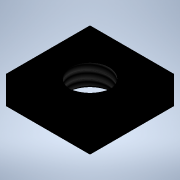
# Autodesk Inventor part: 14122
Saved by Autodesk Inventor 2021 (Build 250183000, 183)
## iProperties
Part Number: 14122
Material: Generic
Catalog Web Link: www.cadenas.de
Description: 14122-Nut
Vendor: 8020
Document SubType Name: Modeling
Designer: partserver
Manufacturer: 8020
Mass: 0.200128 g
Surface Area: 2.76017 cm^2
Volume: 0.200128 cm^3
Density: 1 g/cm^3
Appearance: PSOLRGB-0-0-0
Category: PARTsolutions
Company: 8020
PSOL_IDENT_0: {$CADENAS_DATA\23d-libs\8020\metric\fastening_options\14122.prj},149 {VTYP=3D},{NB=14122},{LINA=1412
PSOL_IDENT_1: 2},{NN=14122},{DATE=31.07.2020 09:21:26},{GEOMDATE=30.03.2012 07:06:00},{VERSION=},{LINEID=10},{WBVA
PSOL_IDENT_2: R=},{WBNUMERIC=}  {NB=14122},{LINA=14122},{KT=DUMMY},{PN=14122},{A=9.000},{B=3.000},{M=5.000}
NB: 14122
NN: 14122
NT: Nut
NBSYN: $PN.
LINA: 14122
CATALOG: 80/20
PN: 14122
A: 9
B: 3
M: 5
SUPPLIER: 8020
ARTICLENO: 14122
BOMINFO: 14122
CREATOR: CADENAS GmbH
Title: 14122
Author: Cadenas PARTsolutions
Comments: Nut
Autodesk Inventor part; units mm, degrees
sketch "Sketch_1" plane through (0, 0, 0) normal (0, 0, 1) x (1, 0, 0)
  line L0 (-4.5, 4.5) -> (-4.5, -4.5)
  line L1 (-4.5, -4.5) -> (4.5, -4.5)
  line L2 (4.5, -4.5) -> (4.5, 4.5)
  line L3 (4.5, 4.5) -> (-4.5, 4.5)
  constraints: 8 end point
extrude "Extrusion1" add sketch "Sketch_1" against normal blind 3
sketch "Sketch_2" plane through (0, 0, 0) normal (1, 0, 0) x (0, 1, 0)
  line L0 (0, -3) -> (0, 0)
  line L1 (0, 0) -> (2.5, 0)
  line L2 (2.5, 0) -> (2.067, -0.433)
  line L3 (2.067, -0.433) -> (2.067, -2.567)
  line L4 (2.067, -2.567) -> (2.5, -3)
  line L5 (2.5, -3) -> (0, -3)
  line L6 (0, -3) -> (0, 0)
  constraints: 14 end point
revolve "Revolution1" cut sketch "Sketch_2" angle 360 about axis through (0, 0, -3) along (0, 0, -1)
thread "Thread1" size "M5x0.8" class "6H" standard "ISO Metric profile" full length
ref_plane "1_XY" through (0, 0, 0) normal (0, 0, 1) x (1, 0, 0)
ref_plane "1_YZ" through (0, 0, 0) normal (1, 0, 0) x (0, 1, 0)
ref_plane "1_ZX" through (0, 0, 0) normal (0, 1, 0) x (0, 0, 1)
body "Solid1"
